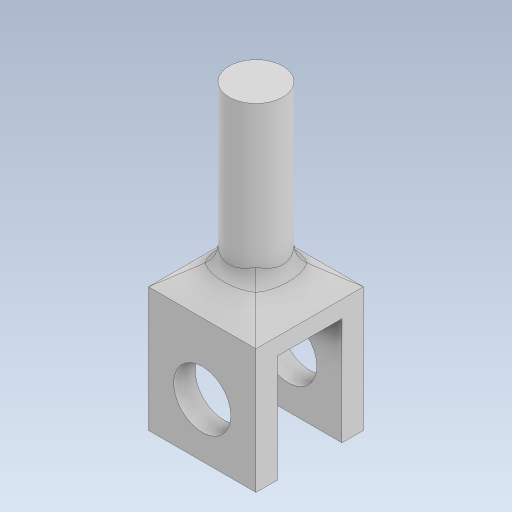
# Autodesk Inventor part: Plunger
Saved by Autodesk Inventor 2023 (Build 270158000, 158)
## iProperties
Created: 2022-09-14
Part Number: Plunger
Material: Generic
Document SubType Name: Modeling
Designer: Dave
Density: 1 g/cm^3
Appearance: Default
Author: Dave
Autodesk Inventor part; units mm, degrees
ref_plane "YZ Plane" through (0, 0, 0) normal (1, 0, 0) x (0, 1, 0)
ref_plane "XZ Plane" through (0, 0, 0) normal (0, 1, 0) x (-1, 0, 0)
sketch "Sketch2" plane through (0, 0, 0) normal (0, 1, 0) x (-1, 0, 0)
  line L0 (6.35, 6.35) -> (-6.35, 6.35)
  line L1 (-6.35, 6.35) -> (-6.35, 3.81)
  line L2 (-6.35, 3.81) -> (6.35, 3.81)
  line L3 (6.35, 3.81) -> (6.35, 6.35)
  line L4 (6.35, -3.81) -> (-6.35, -3.81)
  line L5 (-6.35, -3.81) -> (-6.35, -6.35)
  line L6 (-6.35, -6.35) -> (6.35, -6.35)
  line L7 (6.35, -6.35) -> (6.35, -3.81)
  point P0 (0, 0)
  point P1 (0, 3.81)
  dimension "d0" = 2.54
  dimension "d1" = 7.62
  dimension "d2" = 12.7
  dimension "d23" = 3.81
  constraints: 16 end point, 4 parallel, 2 equal length, 2 horizontal, 2 perpendicular, 1 collinear, 1 midpoint, 1 vertical alignment
  measures "d0" distance of L2.end L0.start
  measures "d1" distance between parallel lines of L2 L4
  measures "d2" distance of L0.start L0.end
  measures "d23" distance from line of L2 point (0, 0)
extrude "Extrusion1" add sketch "Sketch2" along normal blind 12.7
ref_plane "Work Plane1" through (0, 17.7, 0) normal (0, 1, 0) x (1, 0, 0)
sketch "Sketch3" plane through (0, 17.7, 0) normal (0, 1, 0) x (1, 0, 0)
  circle A0 centre (0, 0) radius 3.1825
  line L0 (6.35, -3.81) -> (-6.35, -3.81) projected
  line L1 (-6.35, 3.81) -> (6.35, 3.81) projected
  line L2 (-6.35, -3.81) -> (-6.35, 3.81)
  point P0 (-6.35, 0)
  point P1 (0, -3.81)
  dimension "d6" = 6.365
  constraints: 2 end point, 2 midpoint, 1 centre point, 1 horizontal alignment, 1 vertical, 1 vertical alignment
  measures "d6" diameter of A0
extrude "Extrusion2" add sketch "Sketch3" along normal blind 18
sketch "Sketch4" plane through (0, 12.7, 0) normal (0, 1, 0) x (1, 0, 0)
  line L0 (-6.35, -6.35) -> (6.35, -6.35) projected
  line L1 (6.35, 3.81) -> (6.35, 6.35) projected
  line L2 (-6.35, -6.35) -> (6.35, -6.35)
  line L3 (6.35, -6.35) -> (6.35, 6.35)
  line L4 (6.35, 6.35) -> (-6.35, 6.35)
  line L5 (-6.35, 6.35) -> (-6.35, -6.35)
  point P0 (0, 0)
  constraints: 8 end point, 2 parallel, 1 horizontal, 1 perpendicular
extrude "Extrusion3" add sketch "Sketch4" along normal blind 2
loft "Loft3" add section 1 edges at (0, 14.7, 6.35) (6.35, 14.7, 0) (0, 14.7, -6.35) (-6.35, 14.7, 0) section 2 edges at (-3.1825, 17.7, 0)
sketch "Sketch7" plane through (6.35, 0, -6.35) normal (0, 0, -1) x (-1, 0, 0)
  line L0 (0, 0) -> (0, 12.7) projected
  line L1 (0, 0) -> (12.7, 0) projected
  point P0 (6.35, 0)
  point P1 (6.35, 6.35)
  point P2 (0, 6.35)
  point P3 (6.35, 0)
  constraints: 2 midpoint, 1 horizontal alignment, 1 vertical alignment
hole "Hole1" at (0, 6.35, -6.35) direction (0, 0, 1) diameter 6.7564 end through all clearance for "Flat Head Machine Screw (82)" size "1/4" standard "Ansi Unified Screw Threads"
fillet "Fillet1" radius 2 5 edges at (-3.1825, 17.7, 0) (0, 17.7, -3.1825) (2.9402, 17.7, -1.2179) (0, 17.7, 3.1825) (2.9402, 17.7, 1.2179)
equation "\"d23\" = 0.5 * d1"
body "Solid1"
